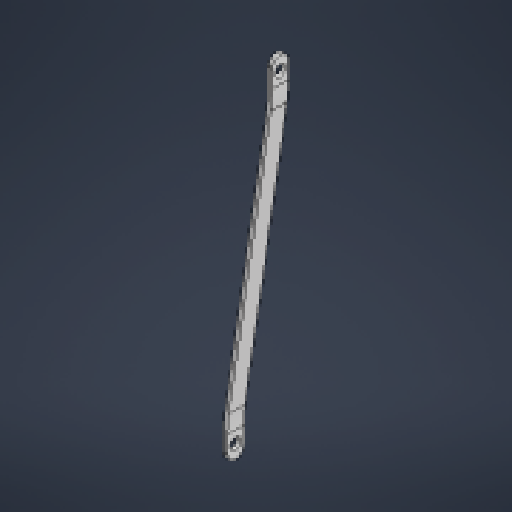
# Autodesk Inventor part: Endgame ramp polycarb
Saved by Autodesk Inventor 2023.2 (Build 272271030, 271C)
## iProperties
Created: 2023-04-06
Part Number: Endgame ramp polycarb
Material: Generic
Document SubType Name: Modeling
Designer: Main Account
Density: 1 g/cm^3
Appearance: Default
Author: Main Account
Autodesk Inventor part; units mm, degrees
ref_plane "YZ Plane" through (0, 0, 0) normal (1, 0, 0) x (0, 1, 0)
ref_plane "XZ Plane" through (0, 0, 0) normal (0, 1, 0) x (-1, 0, 0)
ref_plane "XY Plane" through (0, 0, 0) normal (0, 0, 1) x (1, 0, 0)
sketch "Sketch1" plane through (0, 0, 0) normal (0, 0, 1) x (1, 0, 0)
  line L0 (31.75, 85.8647) -> (31.75, 91.9353) construction
  line L1 (14.2875, -48.6156) -> (14.2875, -52.9844) construction
  line L2 (31.75, 94.2191) -> (31.75, 84.1662)
  line L3 (14.2875, -56.1455) -> (14.2875, -46.0925)
  line L4 (31.2464, 77.0306) -> (14.7911, -38.957)
  arc A0 (31.2464, 77.0306) -> (31.75, 84.1662) centre (-19.05, 84.1662) ccw
  arc A1 (14.7911, -38.957) -> (14.2875, -46.0925) centre (65.0875, -46.0925) ccw
  line L5 (33.3375, 94.2191) -> (33.3375, 84.1662)
  arc A2 (32.8181, 76.8076) -> (33.3375, 84.1662) centre (-19.05, 84.1662) ccw
  line L6 (32.8181, 76.8076) -> (16.3629, -39.1799)
  arc A3 (16.3629, -39.1799) -> (15.875, -46.0925) centre (65.0875, -46.0925) ccw
  line L7 (15.875, -46.0925) -> (15.875, -56.1455)
  line L8 (31.75, 94.2191) -> (33.3375, 94.2191)
  line L9 (14.2875, -56.1455) -> (15.875, -56.1455)
  line L10 (43.5527, 91.6185) -> (43.5527, 89.0199)
  point P0 (0, 0)
  dimension "d0" = 50.8
  dimension "d1" = 50.8
  dimension "d2" = 1.5875
  dimension "d26" = 2.5986
  dimension "d27" = 130.2587
  dimension "d28" = 10.053
  constraints: 18 end point, 8 point on circle, 4 centre point, 4 tangent, 3 vertical, 2 point on line, 1 horizontal, 1 parallel, 1 perpendicular, 4 other
  measures "d0" radius of A0
  measures "d1" radius of A1
  measures "d2" radial gap between concentric circles of A0 A2
  measures "d26" distance of L10.start L10.end
  measures "d27" vertical distance of L7.start L5.end
  measures "d28" distance of L5.start L5.end
extrude "Extrusion1" add sketch "Sketch1" against normal blind 12.7
fillet "Fillet1" radius 6.35 1 edges at (32.5437, 94.2191, 0)
fillet "Fillet2" radius 6.35 1 edges at (32.5437, 94.2191, -12.7)
fillet "Fillet3" radius 6.35 1 edges at (15.0812, -56.1455, 0)
fillet "Fillet4" radius 6.35 1 edges at (15.0812, -56.1455, -12.7)
sketch "Sketch2" plane through (33.3375, 84.1662, 0) normal (1, 0, 0) x (0, 0, -1)
  line L0 (12.7, 10.053) -> (12.7, 0) construction
  line L1 (0, 0) -> (0, 10.053) construction
  line L2 (0, 0) -> (12.7, 0) construction
  circle A0 centre (6.35, 4.7207) radius 6.35
  point P0 (0, -84.1662)
  constraints: 2 tangent, 1 centre point
hole "Hole1" at (33.3375, 88.8868, -6.35) direction (-1, 0, 0) diameter 4.318 end through all
sketch "Sketch3" plane through (15.875, -56.1455, 0) normal (1, 0, 0) x (0, 0, -1)
  line L0 (12.7, 10.053) -> (12.7, 0) construction
  line L1 (0, 0) -> (0, 10.053) construction
  circle A0 centre (6.35, 5.3323) radius 6.35
  line L2 (0, 10.053) -> (12.7, 10.053) construction
  point P0 (0, 56.1455)
  constraints: 2 tangent, 1 centre point
hole "Hole2" at (15.875, -50.8132, -6.35) direction (-1, 0, 0) diameter 4.318 end through all
body "Solid1"
